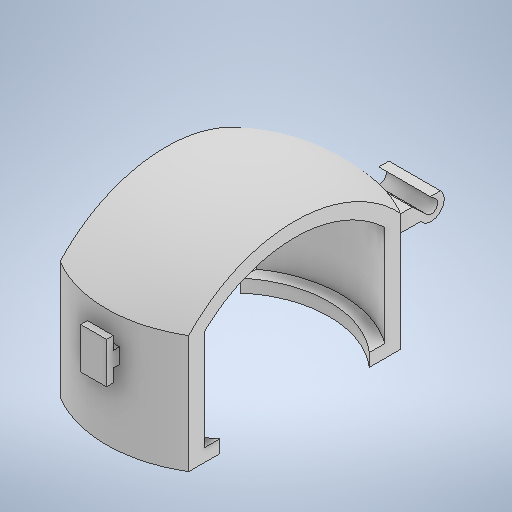
# Autodesk Inventor part: Solar_Panel_Mount
Saved by Autodesk Inventor 2025 (Build 290162010, 162A)
## iProperties
Created: 2024-07-15
Part Number: Solar_Panel_Mount
Material: Generic
Document SubType Name: Modeling
Designer: vncnt
Density: 1 g/cm^3
Appearance: Default
Author: vncnt
Autodesk Inventor part; units mm, degrees
ref_plane "YZ Plane" through (0, 0, 0) normal (1, 0, 0) x (0, 1, 0)
ref_plane "XZ Plane" through (0, 0, 0) normal (0, 1, 0) x (-1, 0, 0)
ref_plane "XY Plane" through (0, 0, 0) normal (0, 0, 1) x (1, 0, 0)
sketch "Sketch3" plane through (0, 0, 0) normal (1, 0, 0) x (0, 1, 0)
  line L0 (24.765, 54.737) -> (-24.765, 54.737)
  line L1 (-24.765, 54.737) -> (-24.765, -54.737)
  line L2 (-24.765, -54.737) -> (24.765, -54.737)
  line L3 (24.765, 54.737) -> (-24.765, -54.737) construction
  line L4 (-24.765, 54.737) -> (24.765, -54.737) construction
  arc A0 (24.765, -54.737) -> (24.765, 54.737) centre (-21.5141, 0) ccw
  line L5 (27.034, 61.087) -> (-31.115, 61.087)
  line L6 (-31.115, 61.087) -> (-31.115, -61.087)
  line L7 (-31.115, -61.087) -> (27.034, -61.087)
  arc A1 (27.034, -61.087) -> (27.034, 61.087) centre (-21.5141, 0) ccw
  line L8 (-38.7767, 48.641) -> (-10.7533, 48.641)
  line L9 (-10.7533, 48.641) -> (-10.7533, -48.641)
  line L10 (-10.7533, -48.641) -> (-38.7767, -48.641)
  line L11 (-38.7767, -48.641) -> (-38.7767, 48.641)
  line L12 (-38.7767, 48.641) -> (-10.7533, -48.641) construction
  line L13 (-10.7533, 48.641) -> (-38.7767, -48.641) construction
  line L14 (-24.765, 0) -> (73.8753, 0)
  point P0 (0, 0)
  point P1 (24.765, 0)
  point P2 (50.165, 0)
  point P3 (50.165, 0)
  point P4 (56.515, 0)
  point P5 (-31.115, 48.641)
  point P6 (-24.765, 48.641)
  dimension "d15" = 63.5
  dimension "d7" = 109.474
  dimension "d9" = 74.93
  dimension "d10" = 49.53
  dimension "d11" = 6.35
  dimension "d13" = 6.096
  constraints: 30 end point, 5 midpoint, 5 point on circle, 4 parallel, 3 horizontal, 3 perpendicular, 2 centre point, 3 other
  measures "d7" distance of L1.end L0.end
  measures "d9" distance of L14.start point (50.165, 0)
  measures "d10" distance of L1.end L2.end
  measures "d11" radial gap between concentric circles of A0 A1
  measures "d13" distance between parallel lines of L10 L2
revolve "Revolution1" add sketch "Sketch3" angle 360 about axis through (0, -24.765, 0) along (0, 1, 0) contours L0 L1 L8 L6 L5 A1 L14 A0
sketch "Sketch4" plane through (0, -31.115, 0) normal (0, -1, 0) x (1, 0, 0)
  line L0 (-31.75, 80.7888) -> (31.75, 80.7888)
  line L1 (31.75, 80.7888) -> (31.75, -80.7888)
  line L2 (31.75, -80.7888) -> (-31.75, -80.7888)
  line L3 (-31.75, -80.7888) -> (-31.75, 80.7888)
  line L4 (-31.75, 80.7888) -> (31.75, -80.7888) construction
  line L5 (31.75, 80.7888) -> (-31.75, -80.7888) construction
  line L6 (64.3082, -113.347) -> (64.3082, 113.347)
  line L7 (64.3082, 113.347) -> (-64.3082, 113.347)
  line L8 (-64.3082, 113.347) -> (-64.3082, -113.347)
  line L9 (-64.3082, -113.347) -> (64.3082, -113.347)
  point P0 (0, 0)
  dimension "d15" = 63.5
  constraints: 20 end point, 4 parallel, 2 midpoint, 2 perpendicular, 1 horizontal, 3 other
  measures "d15" distance of L1.end L2.end
extrude "Extrusion2" cut sketch "Sketch4" against normal through all
sketch "Sketch5" plane through (0, 0, 0) normal (1, 0, 0) x (0, 1, 0)
  line L0 (-31.115, -61.087) -> (27.034, -61.087) projected
  line L1 (-0.4947, -61.087) -> (7.7603, -61.087)
  line L2 (7.7603, -61.087) -> (7.7603, -91.0218)
  line L3 (-0.4947, -81.407) -> (-0.4947, -61.087)
  line L4 (7.7603, -61.087) -> (0.1403, -61.087)
  line L5 (0.1403, -61.087) -> (0.1403, -58.2773)
  line L6 (0.1403, -58.2773) -> (7.7603, -58.2773)
  line L7 (7.7603, -58.2773) -> (7.7603, -61.087)
  arc A0 (1.0316, -84.2813) -> (5.3075, -88.9592) centre (3.3153, -86.487) ccw
  arc A1 (-0.4947, -81.407) -> (9.2585, -84.2506) centre (3.3153, -86.487) ccw
  line L8 (5.3075, -88.9592) -> (9.2585, -84.2506)
  line L9 (5.3075, -88.9592) -> (25.8571, -88.9592) construction
  line L10 (1.0316, -84.2813) -> (2.2156, -92.7411)
  line L11 (7.7603, -77.0191) -> (0.7466, -84.621)
  line L12 (7.7603, -86.487) -> (7.3819, -86.487)
  line L13 (1.3403, -86.487) -> (0.1403, -86.487)
  point P0 (0, 0)
  point P1 (6.0959, -88.0196)
  point P2 (1.7249, -89.2349)
  point P3 (7.7603, -86.036)
  point P4 (1.0353, -84.308)
  dimension "d18" = 7.62
  dimension "d19" = 25.4
  dimension "d20" = 6.35
  dimension "d21" = 12.7
  dimension "d22" = 50
  constraints: 26 end point, 8 point on circle, 5 parallel, 5 point on line, 3 horizontal, 2 centre point, 2 perpendicular, 1 coincident
  measures "d18" distance of L12.start L13.end
  measures "d19" distance of L1.end L12.start
  measures "d20" diameter of A0
  measures "d21" diameter of A1
  measures "d22" angle of L9 L8
extrude "Extrusion3" add sketch "Sketch5" along normal mid plane 25.4 contours L0 L2 L11 L10 A0 A1 L3 | L10 A0 L8 L12 L2 A1 | L2 L12 L8
sketch "Sketch6" plane through (0, 0, 0) normal (1, 0, 0) x (0, 1, 0)
  line L0 (-31.115, 61.087) -> (27.034, 61.087) projected
  line L1 (0, 61.087) -> (20.32, 61.087)
  line L2 (20.32, 61.087) -> (20.32, 67.437)
  line L3 (20.32, 67.437) -> (0, 67.437)
  line L4 (0, 67.437) -> (0, 61.087)
  line L5 (20.32, 61.087) -> (13.97, 61.087)
  line L6 (13.97, 61.087) -> (13.97, 64.135)
  line L7 (13.97, 64.135) -> (20.32, 64.135)
  line L8 (20.32, 64.135) -> (20.32, 61.087)
  line L9 (0, 61.087) -> (6.35, 61.087)
  line L10 (6.35, 61.087) -> (6.35, 64.135)
  line L11 (6.35, 64.135) -> (0, 64.135)
  line L12 (0, 64.135) -> (0, 61.087)
  point P0 (0, 0)
  dimension "d25" = 20.32
  dimension "d26" = 6.35
  dimension "d27" = 6.35
  dimension "d28" = 3.048
  dimension "d29" = 6.35
  dimension "d30" = 3.048
  constraints: 24 end point, 6 parallel, 3 horizontal, 3 perpendicular, 1 point on line
  measures "d25" distance of L3.end L2.end
  measures "d26" distance of L2.end L1.end
  measures "d27" distance of L6.end L7.end
  measures "d28" distance of L5.end L6.end
  measures "d29" distance of L11.end L10.end
  measures "d30" distance of L10.end L9.end
extrude "Extrusion4" add sketch "Sketch6" along normal mid plane 12.7 contours L10 L11 L4 L3 L2 L7 L6 L0
body "Solid2"
